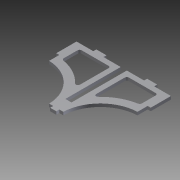
# Autodesk Inventor part: OpenROV 2_2 Aft Ducting Brace
Saved by Autodesk Inventor 2011 (Build 150239000, 239)
## iProperties
Created: 2011-12-01
Part Number: OpenROV 2_2 Aft Ducting Brace
Document SubType Name: Modeling
Designer: user
Density: 1 g/cm^3
Author: user
Autodesk Inventor part; units mm, degrees
ref_plane "YZ Plane" through (0, 0, 0) normal (1, 0, 0) x (0, 1, 0)
ref_plane "XZ Plane" through (0, 0, 0) normal (0, 1, 0) x (-1, 0, 0)
ref_plane "XY Plane" through (0, 0, 0) normal (0, 0, 1) x (1, 0, 0)
sketch "Sketch1" plane through (0, 0, 0) normal (0, 0, 1) x (1, 0, 0)
  line L0 (-46.5, 0) -> (-46.5, -19.95)
  line L1 (-46.5, -19.95) -> (-43.5, -19.95)
  arc A0 (-6.9796, -66.5) -> (-43.5, -29.9796) centre (-45, -68) ccw
  line L2 (-43.5, -19.95) -> (-43.5, -29.9796)
  line L3 (-3, 0) -> (-3, -54.5)
  line L4 (-3, -54.5) -> (0, -54.5)
  line L5 (-20, 0) -> (-20, 3)
  line L6 (-20, 3) -> (-30, 3)
  line L7 (-30, 3) -> (-30, 0)
  line L8 (-46.5, 0) -> (-30, 0)
  line L9 (-20, 0) -> (-3, 0)
  line L10 (-3, -69.5) -> (-3, -66.5)
  line L11 (-38.5, -20.7078) -> (-38.5, -7)
  line L12 (-36.5, -5) -> (-10, -5)
  line L13 (-8, -7) -> (-8, -35.0788)
  arc A1 (-11.4568, -36.4491) -> (-36.8538, -22.6763) centre (-45, -68) ccw
  arc A2 (-38.5, -20.7078) -> (-36.8538, -22.6763) centre (-36.5, -20.7078) ccw
  arc A3 (-36.5, -5) -> (-38.5, -7) centre (-36.5, -7) ccw
  arc A4 (-8, -7) -> (-10, -5) centre (-10, -7) ccw
  arc A5 (-11.4568, -36.4491) -> (-8, -35.0788) centre (-10, -35.0788) ccw
  line L14 (-3, -66.5) -> (-6.9796, -66.5)
  line L15 (-3, -69.5) -> (0, -69.5)
  line L16 (46.5, 0) -> (46.5, -19.95)
  line L17 (46.5, -19.95) -> (43.5, -19.95)
  arc A6 (43.5, -29.9796) -> (6.9796, -66.5) centre (45, -68) ccw
  line L18 (43.5, -19.95) -> (43.5, -29.9796)
  line L19 (3, 0) -> (3, -54.5)
  line L20 (3, -54.5) -> (0, -54.5)
  line L21 (20, 0) -> (20, 3)
  line L22 (20, 3) -> (30, 3)
  line L23 (30, 3) -> (30, 0)
  line L24 (46.5, 0) -> (30, 0)
  line L25 (20, 0) -> (3, 0)
  line L26 (3, -69.5) -> (3, -66.5)
  line L27 (38.5, -20.7078) -> (38.5, -7)
  line L28 (36.5, -5) -> (10, -5)
  line L29 (8, -7) -> (8, -35.0788)
  arc A7 (36.8538, -22.6763) -> (11.4568, -36.4491) centre (45, -68) ccw
  arc A8 (36.8538, -22.6763) -> (38.5, -20.7078) centre (36.5, -20.7078) ccw
  arc A9 (38.5, -7) -> (36.5, -5) centre (36.5, -7) ccw
  arc A10 (10, -5) -> (8, -7) centre (10, -7) ccw
  arc A11 (8, -35.0788) -> (11.4568, -36.4491) centre (10, -35.0788) ccw
  line L30 (3, -66.5) -> (6.9796, -66.5)
  line L31 (3, -69.5) -> (0, -69.5)
  point P0 (0, 0)
  point P1 (-8, -40.5846)
  point P2 (-38.5, -22.411)
  point P3 (8, -40.5846)
  point P4 (38.5, -22.411)
  dimension "d1" = 46.5
  dimension "d3" = 3
  dimension "d5" = 76.1
  dimension "d7" = 45
  dimension "d10" = 10
  dimension "d24" = 10
  dimension "d25" = 20
  dimension "d29" = 3
  dimension "d32" = 8
  dimension "d33" = 5
  dimension "d36" = 17
  dimension "d37" = 16.5
  dimension "d38" = 19.95
  dimension "d39" = 5
  dimension "d40" = 2
  dimension "d45" = 8
  dimension "d49" = 69.5
  dimension "d50" = 15
  constraints: 64 end point, 28 point on circle, 12 centre point, 8 tangent, 6 perpendicular, 4 point on line, 3 equal radius, 3 parallel, 2 coincident
  measures "d1" distance of L0.start point (0, 0)
  measures "d3" distance of L0.end L1.end
  measures "d5" diameter of A0
  measures "d7" horizontal distance of point (0, 0) A0.centre
  measures "d10" distance edge to line of A0 L1
  measures "d24" distance of L5.end L6.end
  measures "d25" distance from line of point (0, 0) L5
  measures "d29" distance of L10.start L10.end
  measures "d32" distance between parallel lines of L0 L11
  measures "d33" distance between parallel lines of L8 L12
  measures "d36" distance of L5.start L3.start
  measures "d37" distance of L0.start L7.end
  measures "d38" distance of L0.start L0.end
  measures "d39" distance between parallel lines of L3 L13
  measures "d40" radius of A2
  measures "d45" radial gap between concentric circles of A0 A1
  measures "d49" distance between parallel lines of L15 L9
  measures "d50" distance between parallel lines of L15 L4
extrude "Extrusion4" add sketch "Sketch1" along normal blind 3
body "Solid4"
